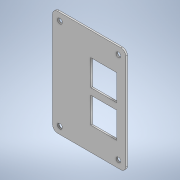
# Autodesk Inventor part: level3_up
Saved by Autodesk Inventor 2021.2 (Build 252289000, 289)
## iProperties
Created: 2021-11-19
Part Number: level3_up
Material: Типовые
Document SubType Name: Modeling
Designer: kanad
Density: 1 g/cm^3
Appearance: По умолчанию
Author: kanad
Autodesk Inventor part; units mm, degrees
ref_plane "YZ Plane" through (0, 0, 0) normal (1, 0, 0) x (0, 1, 0)
ref_plane "XZ Plane" through (0, 0, 0) normal (0, 1, 0) x (-1, 0, 0)
ref_plane "XY Plane" through (0, 0, 0) normal (0, 0, 1) x (1, 0, 0)
sketch "Эскиз1" plane through (0, 0, 0) normal (0, 0, 1) x (1, 0, 0)
  line L0 (1, 18) -> (1, 2) projected
  line L1 (1, 2) -> (17, 2) projected
  line L2 (17, 2) -> (17, 18) projected
  line L3 (17, 18) -> (1, 18) projected
  line L4 (1, -2) -> (1, -18) projected
  line L5 (1, -18) -> (17, -18) projected
  line L6 (17, -18) -> (17, -2) projected
  line L7 (17, -2) -> (1, -2) projected
  line L8 (-22.5, -9) -> (-22.5, -29.5) projected
  arc A0 (-22.5, -29.5) -> (-19.5, -32.5) centre (-19.5, -29.5) ccw projected
  line L9 (-19.5, -32.5) -> (19.5, -32.5) projected
  arc A1 (19.5, -32.5) -> (22.5, -29.5) centre (19.5, -29.5) ccw projected
  line L10 (22.5, -29.5) -> (22.5, 29.5) projected
  arc A2 (22.5, 29.5) -> (19.5, 32.5) centre (19.5, 29.5) ccw projected
  line L11 (19.5, 32.5) -> (-19.5, 32.5) projected
  arc A3 (-19.5, 32.5) -> (-22.5, 29.5) centre (-19.5, 29.5) ccw projected
  line L12 (-22.5, 29.5) -> (-22.5, 9) projected
  line L13 (-22.5, 9) -> (-2, 9) projected
  line L14 (-2, 9) -> (-2, -9) projected
  line L15 (-2, -9) -> (-22.5, -9) projected
  line L16 (1, 18) -> (17, 18) projected
  line L17 (17, 18) -> (17, 2) projected
  line L18 (17, 2) -> (1, 2) projected
  line L19 (1, 2) -> (1, 18) projected
  line L20 (1, -2) -> (17, -2) projected
  line L21 (17, -2) -> (17, -18) projected
  line L22 (17, -18) -> (1, -18) projected
  line L23 (1, -18) -> (1, -2) projected
  circle A4 centre (-18, 28) radius 1.5 projected
  circle A5 centre (18, 28) radius 1.5 projected
  circle A6 centre (18, -28) radius 1.5 projected
  circle A7 centre (-18, -28) radius 1.5 projected
  line L24 (-22.5, 9) -> (-22.5, -9)
  point P0 (0, 0)
  constraints: 2 end point, 1 vertical
extrude "Выдавливание1" add sketch "Эскиз1" along normal blind 1
